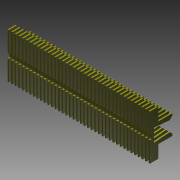
# Autodesk Inventor part: C-229-40-3.00
Saved by Autodesk Inventor 2016 (Build 200138000, 138)
## iProperties
Category: PARTsolutions
Company: SAMTEC
Created: 2016-06-07
Part Number: C-229-40-3.00
Catalog Web Link: www.cadenas.de
Description: C-229-Pins
Vendor: SAMTEC
Document SubType Name: Modeling
Designer: psAdmin
Manufacturer: SAMTEC
Mass: 0.0327562 g
Surface Area: 5.44919 cm^2
Volume: 0.0327562 cm^3
Density: 1 g/cm^3
Material: Generic
Appearance: PSOLRGB-255-255-0
PSOL_IDENT_0: {$CADENAS_DATA\23d-libs\samtec\modelling\ss4\parts\ss4_pins.prj},173 {VTYP=3D},{NB=C-229-40-3.00},{L
PSOL_IDENT_1: INA=C-229-40-3.00},{NN=C-229},{DATE=03.12.2015 13:38:22},{GEOMDATE=03.12.2015 13:33:00},{VERSION=},{
PSOL_IDENT_2: LINEID=10},{LINESUBID=-1},{WBVAR=POS,LS}  {NB=C-229-40-3.00},{LINA=C-229-40-3.00},{KT=DUMMY},{PN=C-2
PSOL_IDENT_3: 29-40-3.00},{SERIES=SS4},{POSALG=   '10' , '-10' , '15' , '-15' , '20' , '-20' , '30' , '-30' ,  '40'
PSOL_IDENT_4: , '-40' , '50' , '-50'   },{POS=40},{LS=3.00},{ROPT=D},{H=3.500},{BH=0.500},{K=2.725},{PINL=5.000},
PSOL_IDENT_5: {PINW=0.150},{PITCH=0.40},{HOLE=0.381},{PINS=40}
NN: C-229
NT: Pins
NB: C-229-40-3.00
NBSYN: $PN.
LINA: C-229-40-3.00
PN: C-229-40-3.00
SERIES: SS4
POS: -40
LS: -3.00
ROPT: D
H: 3.500
BH: 0.500
K: 2.725
PINL: 5.000
PINW: 0.150
PITCH: 0.40
HOLE: 0.381
SUPPLIER: SAMTEC
ARTICLENO: C-229-40-3.00
BOMINFO: C-229-40-3.00
CREATOR: CADENAS GmbH
Title: C-229-40-3.00
Author: Cadenas PARTsolutions
Comments: Pins
Autodesk Inventor part; units mm, degrees
sketch "Sketch_1" plane through (0, 0, 0) normal (1, 0, 0) x (0, 1, 0)
  line L0 (0, 2.5) -> (0, 0.25)
  line L1 (0, 0.25) -> (0.2, 0.25)
  line L2 (0.2, 0.25) -> (0.2, -0.25)
  line L3 (0.2, -0.25) -> (0, -0.25)
  line L4 (0, -0.25) -> (0, -2.5)
  line L5 (0, -2.5) -> (0.85, -2.5)
  arc A0 (0.85, -2.5) -> (0.95, -2.4) centre (0.85, -2.4) ccw
  line L6 (0.95, -2.4) -> (0.95, -1.086)
  line L7 (0.95, -1.086) -> (2.5, -1.086)
  line L8 (2.5, -1.086) -> (2.5, -0.875)
  line L9 (2.5, -0.875) -> (2.2, -0.575)
  line L10 (2.2, -0.575) -> (0.45, -0.7281)
  line L11 (0.45, -0.7281) -> (0.45, 0.7281)
  line L12 (0.45, 0.7281) -> (2.2, 0.575)
  line L13 (2.2, 0.575) -> (2.5, 0.875)
  line L14 (2.5, 0.875) -> (2.5, 1.086)
  line L15 (2.5, 1.086) -> (0.95, 1.086)
  line L16 (0.95, 1.086) -> (0.95, 2.4)
  arc A1 (0.95, 2.4) -> (0.85, 2.5) centre (0.85, 2.4) ccw
  line L17 (0.85, 2.5) -> (0, 2.5)
  constraints: 36 end point, 4 point on circle, 2 centre point
extrude "Extrusion1" add sketch "Sketch_1" along normal mid plane 15.75
sketch "Sketch_3" plane through (0, 0, 0.2) normal (0, 0, 1) x (1, 0, 0)
  line L0 (-7.725, -1.2) -> (7.875, -1.2)
  line L1 (7.875, -1.2) -> (7.875, -1)
  line L2 (7.875, -1) -> (7.725, -1)
  line L3 (7.725, -1) -> (7.725, 3)
  line L4 (7.725, 3) -> (7.475, 3)
  line L5 (7.475, 3) -> (7.475, -1)
  line L6 (7.475, -1) -> (7.325, -1)
  line L7 (7.325, -1) -> (7.325, 3)
  line L8 (7.325, 3) -> (7.075, 3)
  line L9 (7.075, 3) -> (7.075, -1)
  line L10 (7.075, -1) -> (6.925, -1)
  line L11 (6.925, -1) -> (6.925, 3)
  line L12 (6.925, 3) -> (6.675, 3)
  line L13 (6.675, 3) -> (6.675, -1)
  line L14 (6.675, -1) -> (6.525, -1)
  line L15 (6.525, -1) -> (6.525, 3)
  line L16 (6.525, 3) -> (6.275, 3)
  line L17 (6.275, 3) -> (6.275, -1)
  line L18 (6.275, -1) -> (6.125, -1)
  line L19 (6.125, -1) -> (6.125, 3)
  line L20 (6.125, 3) -> (5.875, 3)
  line L21 (5.875, 3) -> (5.875, -1)
  line L22 (5.875, -1) -> (5.725, -1)
  line L23 (5.725, -1) -> (5.725, 3)
  line L24 (5.725, 3) -> (5.475, 3)
  line L25 (5.475, 3) -> (5.475, -1)
  line L26 (5.475, -1) -> (5.325, -1)
  line L27 (5.325, -1) -> (5.325, 3)
  line L28 (5.325, 3) -> (5.075, 3)
  line L29 (5.075, 3) -> (5.075, -1)
  line L30 (5.075, -1) -> (4.925, -1)
  line L31 (4.925, -1) -> (4.925, 3)
  line L32 (4.925, 3) -> (4.675, 3)
  line L33 (4.675, 3) -> (4.675, -1)
  line L34 (4.675, -1) -> (4.525, -1)
  line L35 (4.525, -1) -> (4.525, 3)
  line L36 (4.525, 3) -> (4.275, 3)
  line L37 (4.275, 3) -> (4.275, -1)
  line L38 (4.275, -1) -> (4.125, -1)
  line L39 (4.125, -1) -> (4.125, 3)
  line L40 (4.125, 3) -> (3.875, 3)
  line L41 (3.875, 3) -> (3.875, -1)
  line L42 (3.875, -1) -> (3.725, -1)
  line L43 (3.725, -1) -> (3.725, 3)
  line L44 (3.725, 3) -> (3.475, 3)
  line L45 (3.475, 3) -> (3.475, -1)
  line L46 (3.475, -1) -> (3.325, -1)
  line L47 (3.325, -1) -> (3.325, 3)
  line L48 (3.325, 3) -> (3.075, 3)
  line L49 (3.075, 3) -> (3.075, -1)
  line L50 (3.075, -1) -> (2.925, -1)
  line L51 (2.925, -1) -> (2.925, 3)
  line L52 (2.925, 3) -> (2.675, 3)
  line L53 (2.675, 3) -> (2.675, -1)
  line L54 (2.675, -1) -> (2.525, -1)
  line L55 (2.525, -1) -> (2.525, 3)
  line L56 (2.525, 3) -> (2.275, 3)
  line L57 (2.275, 3) -> (2.275, -1)
  line L58 (2.275, -1) -> (2.125, -1)
  line L59 (2.125, -1) -> (2.125, 3)
  line L60 (2.125, 3) -> (1.875, 3)
  line L61 (1.875, 3) -> (1.875, -1)
  line L62 (1.875, -1) -> (1.725, -1)
  line L63 (1.725, -1) -> (1.725, 3)
  line L64 (1.725, 3) -> (1.475, 3)
  line L65 (1.475, 3) -> (1.475, -1)
  line L66 (1.475, -1) -> (1.325, -1)
  line L67 (1.325, -1) -> (1.325, 3)
  line L68 (1.325, 3) -> (1.075, 3)
  line L69 (1.075, 3) -> (1.075, -1)
  line L70 (1.075, -1) -> (0.925, -1)
  line L71 (0.925, -1) -> (0.925, 3)
  line L72 (0.925, 3) -> (0.675, 3)
  line L73 (0.675, 3) -> (0.675, -1)
  line L74 (0.675, -1) -> (0.525, -1)
  line L75 (0.525, -1) -> (0.525, 3)
  line L76 (0.525, 3) -> (0.275, 3)
  line L77 (0.275, 3) -> (0.275, -1)
  line L78 (0.275, -1) -> (0.125, -1)
  line L79 (0.125, -1) -> (0.125, 3)
  line L80 (0.125, 3) -> (-0.125, 3)
  line L81 (-0.125, 3) -> (-0.125, -1)
  line L82 (-0.125, -1) -> (-0.275, -1)
  line L83 (-0.275, -1) -> (-0.275, 3)
  line L84 (-0.275, 3) -> (-0.525, 3)
  line L85 (-0.525, 3) -> (-0.525, -1)
  line L86 (-0.525, -1) -> (-0.675, -1)
  line L87 (-0.675, -1) -> (-0.675, 3)
  line L88 (-0.675, 3) -> (-0.925, 3)
  line L89 (-0.925, 3) -> (-0.925, -1)
  line L90 (-0.925, -1) -> (-1.075, -1)
  line L91 (-1.075, -1) -> (-1.075, 3)
  line L92 (-1.075, 3) -> (-1.325, 3)
  line L93 (-1.325, 3) -> (-1.325, -1)
  line L94 (-1.325, -1) -> (-1.475, -1)
  line L95 (-1.475, -1) -> (-1.475, 3)
  line L96 (-1.475, 3) -> (-1.725, 3)
  line L97 (-1.725, 3) -> (-1.725, -1)
  line L98 (-1.725, -1) -> (-1.875, -1)
  line L99 (-1.875, -1) -> (-1.875, 3)
  line L100 (-1.875, 3) -> (-2.125, 3)
  line L101 (-2.125, 3) -> (-2.125, -1)
  line L102 (-2.125, -1) -> (-2.275, -1)
  line L103 (-2.275, -1) -> (-2.275, 3)
  line L104 (-2.275, 3) -> (-2.525, 3)
  line L105 (-2.525, 3) -> (-2.525, -1)
  line L106 (-2.525, -1) -> (-2.675, -1)
  line L107 (-2.675, -1) -> (-2.675, 3)
  line L108 (-2.675, 3) -> (-2.925, 3)
  line L109 (-2.925, 3) -> (-2.925, -1)
  line L110 (-2.925, -1) -> (-3.075, -1)
  line L111 (-3.075, -1) -> (-3.075, 3)
  line L112 (-3.075, 3) -> (-3.325, 3)
  line L113 (-3.325, 3) -> (-3.325, -1)
  line L114 (-3.325, -1) -> (-3.475, -1)
  line L115 (-3.475, -1) -> (-3.475, 3)
  line L116 (-3.475, 3) -> (-3.725, 3)
  line L117 (-3.725, 3) -> (-3.725, -1)
  line L118 (-3.725, -1) -> (-3.875, -1)
  line L119 (-3.875, -1) -> (-3.875, 3)
  line L120 (-3.875, 3) -> (-4.125, 3)
  line L121 (-4.125, 3) -> (-4.125, -1)
  line L122 (-4.125, -1) -> (-4.275, -1)
  line L123 (-4.275, -1) -> (-4.275, 3)
  line L124 (-4.275, 3) -> (-4.525, 3)
  line L125 (-4.525, 3) -> (-4.525, -1)
  line L126 (-4.525, -1) -> (-4.675, -1)
  line L127 (-4.675, -1) -> (-4.675, 3)
  line L128 (-4.675, 3) -> (-4.925, 3)
  line L129 (-4.925, 3) -> (-4.925, -1)
  line L130 (-4.925, -1) -> (-5.075, -1)
  line L131 (-5.075, -1) -> (-5.075, 3)
  line L132 (-5.075, 3) -> (-5.325, 3)
  line L133 (-5.325, 3) -> (-5.325, -1)
  line L134 (-5.325, -1) -> (-5.475, -1)
  line L135 (-5.475, -1) -> (-5.475, 3)
  line L136 (-5.475, 3) -> (-5.725, 3)
  line L137 (-5.725, 3) -> (-5.725, -1)
  line L138 (-5.725, -1) -> (-5.875, -1)
  line L139 (-5.875, -1) -> (-5.875, 3)
  line L140 (-5.875, 3) -> (-6.125, 3)
  line L141 (-6.125, 3) -> (-6.125, -1)
  line L142 (-6.125, -1) -> (-6.275, -1)
  line L143 (-6.275, -1) -> (-6.275, 3)
  line L144 (-6.275, 3) -> (-6.525, 3)
  line L145 (-6.525, 3) -> (-6.525, -1)
  line L146 (-6.525, -1) -> (-6.675, -1)
  line L147 (-6.675, -1) -> (-6.675, 3)
  line L148 (-6.675, 3) -> (-6.925, 3)
  line L149 (-6.925, 3) -> (-6.925, -1)
  line L150 (-6.925, -1) -> (-7.075, -1)
  line L151 (-7.075, -1) -> (-7.075, 3)
  line L152 (-7.075, 3) -> (-7.325, 3)
  line L153 (-7.325, 3) -> (-7.325, -1)
  line L154 (-7.325, -1) -> (-7.475, -1)
  line L155 (-7.475, -1) -> (-7.475, 3)
  line L156 (-7.475, 3) -> (-7.725, 3)
  line L157 (-7.725, 3) -> (-7.725, -1.2)
  constraints: 316 end point
extrude "Extrusion2" cut sketch "Sketch_3" along normal blind 3
sketch "Sketch_4" plane through (0, 0, -0.2) normal (0, 0, 1) x (1, 0, 0)
  line L0 (-7.725, -1.2) -> (7.875, -1.2)
  line L1 (7.875, -1.2) -> (7.875, -1)
  line L2 (7.875, -1) -> (7.725, -1)
  line L3 (7.725, -1) -> (7.725, 3)
  line L4 (7.725, 3) -> (7.475, 3)
  line L5 (7.475, 3) -> (7.475, -1)
  line L6 (7.475, -1) -> (7.325, -1)
  line L7 (7.325, -1) -> (7.325, 3)
  line L8 (7.325, 3) -> (7.075, 3)
  line L9 (7.075, 3) -> (7.075, -1)
  line L10 (7.075, -1) -> (6.925, -1)
  line L11 (6.925, -1) -> (6.925, 3)
  line L12 (6.925, 3) -> (6.675, 3)
  line L13 (6.675, 3) -> (6.675, -1)
  line L14 (6.675, -1) -> (6.525, -1)
  line L15 (6.525, -1) -> (6.525, 3)
  line L16 (6.525, 3) -> (6.275, 3)
  line L17 (6.275, 3) -> (6.275, -1)
  line L18 (6.275, -1) -> (6.125, -1)
  line L19 (6.125, -1) -> (6.125, 3)
  line L20 (6.125, 3) -> (5.875, 3)
  line L21 (5.875, 3) -> (5.875, -1)
  line L22 (5.875, -1) -> (5.725, -1)
  line L23 (5.725, -1) -> (5.725, 3)
  line L24 (5.725, 3) -> (5.475, 3)
  line L25 (5.475, 3) -> (5.475, -1)
  line L26 (5.475, -1) -> (5.325, -1)
  line L27 (5.325, -1) -> (5.325, 3)
  line L28 (5.325, 3) -> (5.075, 3)
  line L29 (5.075, 3) -> (5.075, -1)
  line L30 (5.075, -1) -> (4.925, -1)
  line L31 (4.925, -1) -> (4.925, 3)
  line L32 (4.925, 3) -> (4.675, 3)
  line L33 (4.675, 3) -> (4.675, -1)
  line L34 (4.675, -1) -> (4.525, -1)
  line L35 (4.525, -1) -> (4.525, 3)
  line L36 (4.525, 3) -> (4.275, 3)
  line L37 (4.275, 3) -> (4.275, -1)
  line L38 (4.275, -1) -> (4.125, -1)
  line L39 (4.125, -1) -> (4.125, 3)
  line L40 (4.125, 3) -> (3.875, 3)
  line L41 (3.875, 3) -> (3.875, -1)
  line L42 (3.875, -1) -> (3.725, -1)
  line L43 (3.725, -1) -> (3.725, 3)
  line L44 (3.725, 3) -> (3.475, 3)
  line L45 (3.475, 3) -> (3.475, -1)
  line L46 (3.475, -1) -> (3.325, -1)
  line L47 (3.325, -1) -> (3.325, 3)
  line L48 (3.325, 3) -> (3.075, 3)
  line L49 (3.075, 3) -> (3.075, -1)
  line L50 (3.075, -1) -> (2.925, -1)
  line L51 (2.925, -1) -> (2.925, 3)
  line L52 (2.925, 3) -> (2.675, 3)
  line L53 (2.675, 3) -> (2.675, -1)
  line L54 (2.675, -1) -> (2.525, -1)
  line L55 (2.525, -1) -> (2.525, 3)
  line L56 (2.525, 3) -> (2.275, 3)
  line L57 (2.275, 3) -> (2.275, -1)
  line L58 (2.275, -1) -> (2.125, -1)
  line L59 (2.125, -1) -> (2.125, 3)
  line L60 (2.125, 3) -> (1.875, 3)
  line L61 (1.875, 3) -> (1.875, -1)
  line L62 (1.875, -1) -> (1.725, -1)
  line L63 (1.725, -1) -> (1.725, 3)
  line L64 (1.725, 3) -> (1.475, 3)
  line L65 (1.475, 3) -> (1.475, -1)
  line L66 (1.475, -1) -> (1.325, -1)
  line L67 (1.325, -1) -> (1.325, 3)
  line L68 (1.325, 3) -> (1.075, 3)
  line L69 (1.075, 3) -> (1.075, -1)
  line L70 (1.075, -1) -> (0.925, -1)
  line L71 (0.925, -1) -> (0.925, 3)
  line L72 (0.925, 3) -> (0.675, 3)
  line L73 (0.675, 3) -> (0.675, -1)
  line L74 (0.675, -1) -> (0.525, -1)
  line L75 (0.525, -1) -> (0.525, 3)
  line L76 (0.525, 3) -> (0.275, 3)
  line L77 (0.275, 3) -> (0.275, -1)
  line L78 (0.275, -1) -> (0.125, -1)
  line L79 (0.125, -1) -> (0.125, 3)
  line L80 (0.125, 3) -> (-0.125, 3)
  line L81 (-0.125, 3) -> (-0.125, -1)
  line L82 (-0.125, -1) -> (-0.275, -1)
  line L83 (-0.275, -1) -> (-0.275, 3)
  line L84 (-0.275, 3) -> (-0.525, 3)
  line L85 (-0.525, 3) -> (-0.525, -1)
  line L86 (-0.525, -1) -> (-0.675, -1)
  line L87 (-0.675, -1) -> (-0.675, 3)
  line L88 (-0.675, 3) -> (-0.925, 3)
  line L89 (-0.925, 3) -> (-0.925, -1)
  line L90 (-0.925, -1) -> (-1.075, -1)
  line L91 (-1.075, -1) -> (-1.075, 3)
  line L92 (-1.075, 3) -> (-1.325, 3)
  line L93 (-1.325, 3) -> (-1.325, -1)
  line L94 (-1.325, -1) -> (-1.475, -1)
  line L95 (-1.475, -1) -> (-1.475, 3)
  line L96 (-1.475, 3) -> (-1.725, 3)
  line L97 (-1.725, 3) -> (-1.725, -1)
  line L98 (-1.725, -1) -> (-1.875, -1)
  line L99 (-1.875, -1) -> (-1.875, 3)
  line L100 (-1.875, 3) -> (-2.125, 3)
  line L101 (-2.125, 3) -> (-2.125, -1)
  line L102 (-2.125, -1) -> (-2.275, -1)
  line L103 (-2.275, -1) -> (-2.275, 3)
  line L104 (-2.275, 3) -> (-2.525, 3)
  line L105 (-2.525, 3) -> (-2.525, -1)
  line L106 (-2.525, -1) -> (-2.675, -1)
  line L107 (-2.675, -1) -> (-2.675, 3)
  line L108 (-2.675, 3) -> (-2.925, 3)
  line L109 (-2.925, 3) -> (-2.925, -1)
  line L110 (-2.925, -1) -> (-3.075, -1)
  line L111 (-3.075, -1) -> (-3.075, 3)
  line L112 (-3.075, 3) -> (-3.325, 3)
  line L113 (-3.325, 3) -> (-3.325, -1)
  line L114 (-3.325, -1) -> (-3.475, -1)
  line L115 (-3.475, -1) -> (-3.475, 3)
  line L116 (-3.475, 3) -> (-3.725, 3)
  line L117 (-3.725, 3) -> (-3.725, -1)
  line L118 (-3.725, -1) -> (-3.875, -1)
  line L119 (-3.875, -1) -> (-3.875, 3)
  line L120 (-3.875, 3) -> (-4.125, 3)
  line L121 (-4.125, 3) -> (-4.125, -1)
  line L122 (-4.125, -1) -> (-4.275, -1)
  line L123 (-4.275, -1) -> (-4.275, 3)
  line L124 (-4.275, 3) -> (-4.525, 3)
  line L125 (-4.525, 3) -> (-4.525, -1)
  line L126 (-4.525, -1) -> (-4.675, -1)
  line L127 (-4.675, -1) -> (-4.675, 3)
  line L128 (-4.675, 3) -> (-4.925, 3)
  line L129 (-4.925, 3) -> (-4.925, -1)
  line L130 (-4.925, -1) -> (-5.075, -1)
  line L131 (-5.075, -1) -> (-5.075, 3)
  line L132 (-5.075, 3) -> (-5.325, 3)
  line L133 (-5.325, 3) -> (-5.325, -1)
  line L134 (-5.325, -1) -> (-5.475, -1)
  line L135 (-5.475, -1) -> (-5.475, 3)
  line L136 (-5.475, 3) -> (-5.725, 3)
  line L137 (-5.725, 3) -> (-5.725, -1)
  line L138 (-5.725, -1) -> (-5.875, -1)
  line L139 (-5.875, -1) -> (-5.875, 3)
  line L140 (-5.875, 3) -> (-6.125, 3)
  line L141 (-6.125, 3) -> (-6.125, -1)
  line L142 (-6.125, -1) -> (-6.275, -1)
  line L143 (-6.275, -1) -> (-6.275, 3)
  line L144 (-6.275, 3) -> (-6.525, 3)
  line L145 (-6.525, 3) -> (-6.525, -1)
  line L146 (-6.525, -1) -> (-6.675, -1)
  line L147 (-6.675, -1) -> (-6.675, 3)
  line L148 (-6.675, 3) -> (-6.925, 3)
  line L149 (-6.925, 3) -> (-6.925, -1)
  line L150 (-6.925, -1) -> (-7.075, -1)
  line L151 (-7.075, -1) -> (-7.075, 3)
  line L152 (-7.075, 3) -> (-7.325, 3)
  line L153 (-7.325, 3) -> (-7.325, -1)
  line L154 (-7.325, -1) -> (-7.475, -1)
  line L155 (-7.475, -1) -> (-7.475, 3)
  line L156 (-7.475, 3) -> (-7.725, 3)
  line L157 (-7.725, 3) -> (-7.725, -1.2)
  constraints: 316 end point
extrude "Extrusion3" cut sketch "Sketch_4" against normal blind 3
ref_plane "pins_to_socket_XY" through (0, 0, 0) normal (0, 1, 0) x (1, 0, 0)
ref_plane "pins_to_socket_YZ" through (0, 0, 0) normal (1, 0, 0) x (0, 0, -1)
ref_plane "pins_to_socket_ZX" through (0, 0, 0) normal (0, 0, -1) x (0, 1, 0)
body "Solid1"
